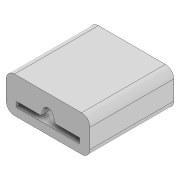
# Autodesk Inventor part: Cable_tie_attachment
Saved by Autodesk Inventor 2022 (Build 260153000, 153)
## iProperties
Created: 2022-08-29
Part Number: Cable_tie_attachment
Material: Generic
Document SubType Name: Modeling
Designer: dell
Density: 1 g/cm^3
Appearance: Default
Author: dell
Autodesk Inventor part; units mm, degrees
ref_plane "YZ Plane" through (0, 0, 0) normal (1, 0, 0) x (0, 1, 0)
ref_plane "XZ Plane" through (0, 0, 0) normal (0, 1, 0) x (-1, 0, 0)
ref_plane "XY Plane" through (0, 0, 0) normal (0, 0, 1) x (1, 0, 0)
sketch "Sketch1" plane through (0, 0, 0) normal (0, 0, 1) x (1, 0, 0)
  line L0 (-5, 0) -> (5, 0)
  line L1 (5, 0) -> (5, 4.3)
  line L2 (5, 4.3) -> (-5, 4.3)
  line L3 (-5, 4.3) -> (-5, 0)
  line L4 (-3.75, 0) -> (3.75, 0)
  line L5 (3.75, 0) -> (3.75, 1.6)
  line L6 (3.75, 1.6) -> (-3.75, 1.6)
  line L7 (-3.75, 1.6) -> (-3.75, 0)
  line L8 (-3.75, 1) -> (3.75, 1)
  circle A0 centre (0, 2.2) radius 0.6
  line L9 (-0.5638, 2.4052) -> (-0.8569, 1.6)
  line L10 (0.5638, 2.4052) -> (0.8569, 1.6)
  point P0 (0, 0)
  dimension "d0" = 10
  dimension "d1" = 7.5
  dimension "d2" = 3.75
  dimension "d3" = 5
  dimension "d4" = 1
  dimension "d5" = 0.6
  dimension "d6" = 1.2
  dimension "d7" = 1.5
  dimension "d8" = 70
  dimension "d9" = 70
  constraints: 22 end point, 5 point on line, 4 parallel, 3 perpendicular, 3 tangent, 2 horizontal, 2 point on circle, 1 centre point, 1 midpoint
  measures "d0" distance of L0.start L0.end
  measures "d1" distance between parallel lines of L7 L5
  measures "d2" distance from line of point (0, 0) L7
  measures "d3" distance from line of point (0, 0) L3
  measures "d4" distance between parallel lines of L0 L8
  measures "d5" distance between parallel lines of L6 L8
  measures "d6" diameter of A0
  measures "d7" distance edge to line of A0 L2
  measures "d8" angle of L6 L9
  measures "d9" angle of L6 L10
extrude "Extrusion1" add sketch "Sketch1" along normal blind 10 contours L3 L2 L1 L0 L5 L6 L10 A0 L9 L7 | L7 L8 L5 L0
fillet "Fillet1" radius 1 4 edges at (5, 4.3, 5) (5, 0, 5) (-5, 4.3, 5) (-5, 0, 5)
equation "\"d2\" = 0.5 * d1"
equation "\"d3\" = 0.5 * d0"
body "Solid1"
